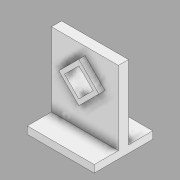
# Autodesk Inventor part: base_end_mounts
Saved by Autodesk Inventor 2020 (Build 240168000, 168)
## iProperties
Created: 2021-04-02
Part Number: base_end_mounts
Material: ABS Plastic
Document SubType Name: Modeling
Designer: griss
Density: 1.06 g/cm^3
Appearance: Smooth - White
Author: griss
Autodesk Inventor part; units mm, degrees
ref_plane "YZ Plane" through (0, 0, 0) normal (1, 0, 0) x (0, 1, 0)
ref_plane "XZ Plane" through (0, 0, 0) normal (0, 1, 0) x (-1, 0, 0)
ref_plane "XY Plane" through (0, 0, 0) normal (0, 0, 1) x (1, 0, 0)
sketch "Sketch1" plane through (0, 0, 0) normal (0, 0, 1) x (1, 0, 0)
  line L0 (0, 17.9605) -> (17.9605, 0) construction
  line L1 (17.9605, 0) -> (0, -17.9605) construction
  line L2 (0, -17.9605) -> (-17.9605, 0) construction
  line L3 (-17.9605, 0) -> (0, 17.9605) construction
  line L4 (0, 17.9605) -> (0, -17.9605) construction
  line L5 (17.9605, 0) -> (-17.9605, 0) construction
  line L6 (0, 17.9605) -> (-17.9605, 0)
  line L7 (0, -86.3372) -> (0, 55.9028) projected
  line L8 (-58.674, 0) -> (58.674, 0) projected
  line L9 (0, 17.9605) -> (17.9605, 0)
  line L10 (17.9605, 0) -> (0, -17.9605)
  line L11 (-17.9605, 0) -> (0, -17.9605)
  line L12 (0, 25.1447) -> (-25.1447, 0)
  line L13 (-25.1447, 0) -> (0, -25.1447)
  line L14 (0, -25.1447) -> (25.1447, 0)
  line L15 (25.1447, 0) -> (0, 25.1447)
  line L16 (-41.91, 35.5828) -> (41.91, 35.5828)
  line L17 (41.91, 35.5828) -> (41.91, -66.0172)
  line L18 (41.91, -66.0172) -> (-41.91, -66.0172)
  line L19 (-41.91, -66.0172) -> (-41.91, 35.5828)
  point P0 (0, 0)
  point P1 (0, 0)
  point P2 (0, 0)
  point P3 (0, 0)
  point P4 (0, 0)
  point P5 (29.7157, 21.8287)
  point P6 (0, 35.5828)
  dimension "d0" = 25.4
  dimension "d1" = 25.4
  dimension "d5" = 0
  dimension "d6" = 5.08
  dimension "d7" = 5.08
  dimension "d15" = 83.82
  dimension "d16" = 101.6
  constraints: 36 end point, 10 perpendicular, 5 midpoint, 3 coincident, 2 parallel, 1 horizontal, 1 horizontal alignment, 1 point on line, 1 vertical alignment, 8 other
  measures "d0" distance of L1.end L2.end
  measures "d1" distance of L0.end L1.end
  measures "d5" distance between parallel lines of L9 L0
  measures "d6" distance between parallel lines of L12 L6
  measures "d7" distance between parallel lines of L11 L13
  measures "d15" distance of L16.start L16.end
  measures "d16" distance of L16.end L17.end
extrude "Extrusion2" add sketch "Sketch1" along normal blind 20.32 contours L6 L8 L12 L7 | L7 L15 L8 L9 | L11 L7 L13 L8 | L8 L14 L7 L10
extrude "Extrusion3" add sketch "Sketch1" along normal blind 12.7 contours L12 L8 L19 L16 L7 | L7 L16 L17 L8 L15 | L13 L7 L18 L19 L8 | L8 L17 L18 L7 L14
sketch "Sketch2" plane through (41.91, -66.0172, 0) normal (1, 0, 0) x (0, 0, -1)
  line L0 (0, 0) -> (0, 101.6) projected
  line L1 (0, 101.6) -> (-12.7, 101.6) projected
  line L2 (-12.7, 0) -> (-12.7, 101.6) projected
  line L3 (0, 0) -> (-12.7, 0) projected
  line L4 (-42.9388, 0) -> (30.2388, 0)
  line L5 (30.2388, 0) -> (30.2388, 9.2066)
  line L6 (30.2388, 9.2066) -> (-42.9388, 9.2066)
  line L7 (-42.9388, 9.2066) -> (-42.9388, 0)
  line L8 (-42.9388, 0) -> (30.2388, 9.2066) construction
  line L9 (30.2388, 0) -> (-42.9388, 9.2066) construction
  point P0 (0, 66.0172)
  point P1 (-6.35, 4.6033)
  point P2 (-6.35, 0)
  constraints: 12 end point, 4 midpoint, 2 parallel, 1 horizontal, 1 perpendicular
extrude "Extrusion4" add sketch "Sketch2" against normal up to surface (83.82 mm away) contours L3 L2 L6 L0 | L0 L6 L5 L4 | L4 L7 L6 L2
equation "\"d7\" = d6"
body "Solid1"
